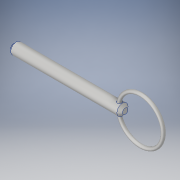
# Autodesk Inventor part: Release_Pin
Saved by Autodesk Inventor 2019 (Build 230136000, 136)
## iProperties
Created: 2021-01-31
Part Number: Release_Pin
Material: Aluminum 6061
Document SubType Name: Modeling
Designer: zhanb
Density: 2.7 g/cm^3
Appearance: Aluminum - Flat
Author: zhanb
Autodesk Inventor part; units mm, degrees
ref_plane "YZ Plane" through (0, 0, 0) normal (1, 0, 0) x (0, 1, 0)
ref_plane "XZ Plane" through (0, 0, 0) normal (0, 1, 0) x (-1, 0, 0)
ref_plane "XY Plane" through (0, 0, 0) normal (0, 0, 1) x (1, 0, 0)
sketch "Sketch1" plane through (0, 0, 0) normal (1, 0, 0) x (0, 1, 0)
  circle A0 centre (0, 0) radius 3.175
  dimension "d0" = 6.35
  constraints: 1 centre point, 1 coincident
  measures "d0" diameter of A0
extrude "Extrusion1" add sketch "Sketch1" along normal mid plane 63.5
sketch "Sketch2" plane through (0, 0, 0) normal (0, 1, 0) x (-1, 0, 0)
  circle A0 centre (-28.575, 0) radius 1.27
  line L0 (-31.75, 3.175) -> (-31.75, -3.175) projected
  point P0 (0, 0)
  dimension "d3" = 2.54
  dimension "d4" = 3.175
  constraints: 1 centre point
  measures "d3" diameter of A0
  measures "d4" distance from line of L0 A0.centre
extrude "Extrusion2" cut sketch "Sketch2" along normal through all both and the other way through all
sketch "Sketch3" plane through (0, 0, 0) normal (0, 0, 1) x (1, 0, 0)
  circle A0 centre (40.64, 0) radius 12.7
  point P0 (0, 0)
  dimension "d7" = 25.4
  dimension "d8" = 40.64
  constraints: 1 centre point, 1 horizontal alignment
  measures "d7" diameter of A0
  measures "d8" distance of A0.centre point (0, 0)
sketch "Sketch4" plane through (0, 0, 0) normal (0, 1, 0) x (-1, 0, 0)
  line L0 (-27.94, 0) -> (-53.34, 0) construction
  circle A0 centre (-53.34, 0) radius 1.016
  point P0 (0, 0)
  dimension "d9" = 2.032
  constraints: 2 coincident, 1 centre point
  measures "d9" diameter of A0
sweep "Sweep1" add profiles "Sketch4" path "Sketch3"
sketch "Sketch5" plane through (0, 0, 0) normal (0, 1, 0) x (-1, 0, 0)
  line L0 (28.575, 0) -> (28.575, -3.9688)
  arc A0 (26.9875, -2.3813) -> (28.575, -3.9688) centre (28.575, -2.3813) ccw
  line L1 (26.9875, -2.3813) -> (26.9875, 0)
  line L2 (26.9875, 0) -> (28.575, 0)
  line L3 (31.75, -3.175) -> (31.75, 3.175) projected
  point P0 (0, 0)
  dimension "d12" = 1.5875
  dimension "d13" = 3.175
  dimension "d14" = 0.7937
  constraints: 6 end point, 2 point on circle, 2 vertical, 1 centre point, 1 horizontal alignment, 1 perpendicular, 1 point on line, 1 tangent
  measures "d12" radius of A0
  measures "d13" distance from line of L3 L0.start
  measures "d14" vertical distance of L3.start A0.centre
revolve "Revolution1" add sketch "Sketch5" angle 360 about axis through (-28.575, 0, 0) along (0, 0, -1)
chamfer "Chamfer1" distance 1.5875 angle 45 2 edges at (-31.75, -3.175, 0) (31.75, -3.175, 0)
body "Solid1"
